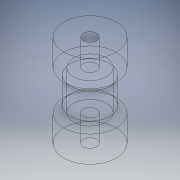
# Autodesk Inventor part: 기본 투상 연습4
Saved by Autodesk Inventor 2018.3 (Build 223284000, 284)
## iProperties
Created: 2019-10-08
Part Number: 기본 투상 연습4
Material: 일반
Document SubType Name: Modeling
Designer: MyTool
Density: 1 g/cm^3
Appearance: 기본값
Author: MyTool
Autodesk Inventor part; units mm, degrees
ref_plane "YZ Plane" through (0, 0, 0) normal (1, 0, 0) x (0, 1, 0)
ref_plane "XZ Plane" through (0, 0, 0) normal (0, 1, 0) x (-1, 0, 0)
ref_plane "XY Plane" through (0, 0, 0) normal (0, 0, 1) x (1, 0, 0)
sketch "스케치4" plane through (0, 0, 0) normal (1, 0, 0) x (0, 1, 0)
  line L0 (0, 0) -> (0, 70)
  line L1 (0, 70) -> (20, 70)
  line L2 (20, 70) -> (20, 50)
  line L3 (20, 50) -> (15, 45)
  line L4 (15, 45) -> (15, 25)
  line L5 (15, 25) -> (20, 20)
  line L6 (20, 20) -> (20, 0)
  line L7 (20, 0) -> (0, 0)
  dimension "d98" = 70
  dimension "d99" = 20
  dimension "d100" = 20
  dimension "d101" = 20
  dimension "d102" = 20
  dimension "d103" = 5
  dimension "d104" = 5
  constraints: 16 end point, 3 perpendicular, 2 point on line, 1 parallel, 1 vertical
  measures "d98" distance of L0.start L0.end
  measures "d99" distance of L0.end L1.end
  measures "d100" distance of L1.end L2.end
  measures "d101" distance of L3.end L4.end
  measures "d102" distance of L5.end L6.end
  measures "d103" horizontal distance of L4.end L5.end
  measures "d104" horizontal distance of L2.end L3.end
revolve "회전2" add sketch "스케치4" angle 360 about axis through (0, 0, 0) along (0, 0, 1)
sketch "스케치5" plane through (0, 0, 70) normal (0, 0, 1) x (1, 0, 0)
  circle A0 centre (0, 0) radius 5
  dimension "d106" = 10
  constraints: 1 centre point, 1 coincident
  measures "d106" diameter of A0
extrude "돌출1" cut sketch "스케치5" against normal blind 20
sketch "스케치6" plane through (0, 0, 50) normal (0, 0, 1) x (1, 0, 0)
  circle A0 centre (0, 0) radius 12.5
  dimension "d109" = 25
  constraints: 1 centre point, 1 coincident
  measures "d109" diameter of A0
extrude "돌출2" cut sketch "스케치6" against normal blind 30
sketch "스케치7" plane through (0, 0, 20) normal (0, 0, 1) x (1, 0, 0)
  circle A0 centre (0, 0) radius 5
  dimension "d112" = 10
  constraints: 1 centre point, 1 coincident
  measures "d112" diameter of A0
extrude "돌출3" cut sketch "스케치7" against normal up to next
